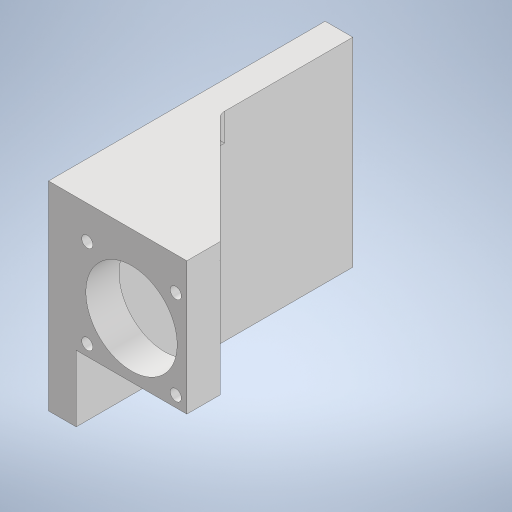
# Autodesk Inventor part: Z_motor_holder
Saved by Autodesk Inventor 2024.1 (Build 281209000, 209)
## iProperties
Created: 2023-09-27
Part Number: Z_motor_holder
Material: Generic
Document SubType Name: Modeling
Designer: l1534
Density: 1 g/cm^3
Appearance: Default
Author: l1534
Autodesk Inventor part; units mm, degrees
ref_plane "YZ Plane" through (0, 0, 0) normal (1, 0, 0) x (0, 1, 0)
ref_plane "XZ Plane" through (0, 0, 0) normal (0, 1, 0) x (-1, 0, 0)
ref_plane "XY Plane" through (0, 0, 0) normal (0, 0, 1) x (1, 0, 0)
sketch "Sketch1" plane through (0, 0, 0) normal (1, 0, 0) x (0, 1, 0)
  line L0 (-23.3447, 18.3788) -> (12.6553, 18.3788)
  line L1 (12.6553, 18.3788) -> (12.6553, -31.6212)
  line L2 (12.6553, -31.6212) -> (-23.3447, -31.6212)
  line L3 (-23.3447, -31.6212) -> (-23.3447, 18.3788)
  point P0 (0, 0)
  dimension "d0" = 36
  dimension "d1" = 50
  constraints: 8 end point, 2 parallel, 1 horizontal, 1 perpendicular
  measures "d0" distance of L0.start L0.end
  measures "d1" distance of L2.end L0.start
extrude "Extrusion1" add sketch "Sketch1" along normal blind 5
sketch "Sketch2" plane through (5, 0, 0) normal (1, 0, 0) x (0, 0, -1)
  line L0 (31.6212, 12.6553) -> (-18.3788, 12.6553) projected
  line L1 (-18.3788, 12.6553) -> (-12.3788, 12.6553)
  line L2 (-12.3788, 12.6553) -> (-12.3788, -11.3447)
  line L3 (-12.3788, -11.3447) -> (-18.3788, -11.3447)
  line L4 (-18.3788, -11.3447) -> (-18.3788, 12.6553)
  point P0 (0, 0)
  dimension "d4" = 24
  dimension "d5" = 6
  constraints: 8 end point, 2 parallel, 1 horizontal, 1 perpendicular
  measures "d4" distance of L3.end L0.end
  measures "d5" distance of L2.end L3.end
extrude "Extrusion2" add sketch "Sketch2" along normal blind 20
sketch "Sketch3" plane through (5, -11.3447, 12.3788) normal (0, 0, -1) x (-1, 0, 0)
  circle A0 centre (-10, 10) radius 8.25
  line L0 (-20, 0) -> (-20, 24) projected
  line L1 (0, 0) -> (-20, 0) projected
  circle A1 centre (-18, 2) radius 1
  circle A2 centre (-18, 18) radius 1
  circle A3 centre (-2, 2) radius 1
  circle A4 centre (-2, 18) radius 1
  point P0 (5, 11.3447)
  dimension "d8" = 16.5
  dimension "d9" = 10
  dimension "d10" = 10
  dimension "d11" = 2
  dimension "d12" = 2
  dimension "d13" = 2
  dimension "d14" = 2
  dimension "d15" = 8
  dimension "d16" = 8
  dimension "d17" = 8
  dimension "d18" = 8
  dimension "d19" = 8
  dimension "d20" = 8
  dimension "d21" = 8
  dimension "d22" = 8
  constraints: 5 centre point
  measures "d8" diameter of A0
  measures "d9" distance from line of L0 A0.centre
  measures "d10" distance from line of L1 A0.centre
  measures "d11" diameter of A1
  measures "d12" diameter of A2
  measures "d13" diameter of A3
  measures "d14" diameter of A4
  measures "d15" horizontal distance of A0.centre A1.centre
  measures "d16" horizontal distance of A0.centre A1.centre
  measures "d17" horizontal distance of A0.centre A2.centre
  measures "d18" horizontal distance of A0.centre A2.centre
  measures "d19" horizontal distance of A0.centre A3.centre
  measures "d20" horizontal distance of A0.centre A3.centre
  measures "d21" horizontal distance of A0.centre A4.centre
  measures "d22" horizontal distance of A0.centre A4.centre
extrude "Extrusion3" cut sketch "Sketch3" against normal through all
sketch "Sketch4" plane through (5, -11.3447, 12.3788) normal (0, 0, -1) x (-1, 0, 0)
  line L0 (-20, 24) -> (-20, 0) projected
  line L1 (0, 24) -> (0, 0) projected
  line L2 (-20, 24) -> (0, 24)
  line L3 (0, 24) -> (0, 21)
  line L4 (0, 21) -> (-20, 21)
  line L5 (-20, 21) -> (-20, 24)
  point P0 (5, 11.3447)
  dimension "d25" = 3
  constraints: 8 end point, 2 parallel, 1 horizontal, 1 perpendicular, 1 point on line
  measures "d25" distance between parallel lines of L2 L4
extrude "Extrusion4" add sketch "Sketch4" along normal blind 20
sketch "Sketch5" plane through (5, 9.6553, 12.3788) normal (0, -1, 0) x (1, 0, 0)
  line L0 (0, -20) -> (0, 0) projected
  line L1 (20, 6) -> (20, 0) projected
  line L2 (0, -20) -> (20, 0)
  line L3 (20, 0) -> (20, -20)
  line L4 (20, -20) -> (0, -20) projected
  line L5 (20, -20) -> (0, -20)
  point P0 (-5, -12.3788)
  constraints: 6 end point, 2 collinear
extrude "Extrusion5" cut sketch "Sketch5" against normal through all
fillet "Fillet1" radius 2 2 edges at (5, 9.6553, 2.3788) (5, 11.1553, -7.6212)
body "Solid1"
